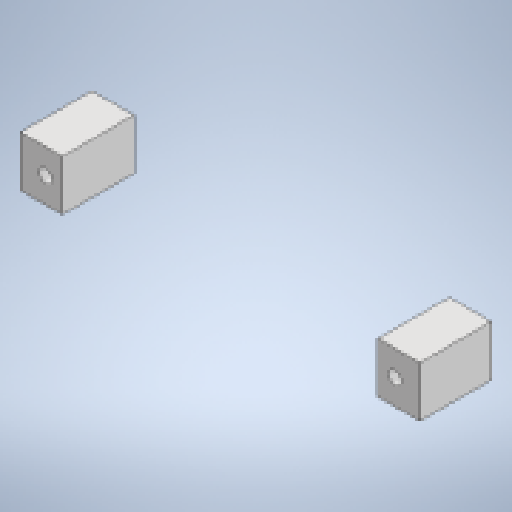
# Autodesk Inventor part: Tapadera cremallera
Saved by Autodesk Inventor 2024 (Build 280153000, 153)
## iProperties
Created: 2025-03-05
Part Number: Tapadera cremallera
Material: Genérico
Document SubType Name: Modeling
Designer: sergi
Density: 1 g/cm^3
Appearance: Valor por defecto
Author: sergi
Autodesk Inventor part; units mm, degrees
ref_plane "YZ Plane" through (0, 0, 0) normal (1, 0, 0) x (0, 1, 0)
ref_plane "XZ Plane" through (0, 0, 0) normal (0, 1, 0) x (-1, 0, 0)
sketch "Boceto1" plane through (0, 0, 0) normal (0, 0, 1) x (1, 0, 0)
  line L0 (9.8963, 1.0011) -> (-9.8944, 1.0011) projected
  arc A0 (-33.0611, -12.6806) -> (-9.8944, 1.0011) centre (-23.4499, -2.5004) ccw projected
  line L1 (-33.0611, -12.6806) -> (-33.2, -12.6806) projected
  line L2 (-33.2, -12.6806) -> (-33.2, -12.5477) projected
  arc A1 (-37.0054, 1.0011) -> (-33.2, -12.5477) centre (-23.4499, -2.5004) ccw projected
  line L3 (-37.0054, 1.0011) -> (-47.5, 1.0011) projected
  line L4 (-47.5, 1.0011) -> (-47.5, -20) projected
  line L5 (-47.5, -20) -> (47.5, -20) projected
  line L6 (47.5, -20) -> (47.5, 1.0011) projected
  line L7 (47.5, 1.0011) -> (37.0052, 1.0011) projected
  arc A2 (33.2, -12.5466) -> (37.0052, 1.0011) centre (23.4507, -2.5001) ccw projected
  line L8 (33.2, -12.5466) -> (33.2, -12.6806) projected
  line L9 (33.2, -12.6806) -> (33.06, -12.6806) projected
  arc A3 (9.8963, 1.0011) -> (33.06, -12.6806) centre (23.4507, -2.5001) ccw projected
  circle A4 centre (40.9504, -2.4989) radius 2.1 projected
  circle A5 centre (5.9501, -2.5002) radius 2.1 projected
  circle A6 centre (-5.9495, -2.4989) radius 2.1 projected
  circle A7 centre (-40.9494, -2.4994) radius 2.1 projected
  line L10 (47.5, -20) -> (41.5, -20)
  line L11 (41.5, -20) -> (41.5, -14)
  line L12 (41.5, -14) -> (47.5, -14)
  line L13 (47.5, -14) -> (47.5, -20)
  circle A8 centre (41.5, -14) radius 1.6
  line L14 (-47.5, -20) -> (-41.5, -20)
  line L15 (-41.5, -20) -> (-41.5, -14)
  line L16 (-41.5, -14) -> (-47.5, -14)
  line L17 (-47.5, -14) -> (-47.5, -20)
  circle A9 centre (-41.5, -14) radius 1.6
  line L18 (47.5, -20) -> (33.5, -20)
  line L19 (33.5, -20) -> (33.5, -8)
  line L20 (33.5, -8) -> (47.5, -8)
  line L21 (47.5, -8) -> (47.5, -20)
  line L22 (-47.5, -20) -> (-33.5, -20)
  line L23 (-33.5, -20) -> (-33.5, -8)
  line L24 (-33.5, -8) -> (-47.5, -8)
  line L25 (-47.5, -8) -> (-47.5, -20)
  line L26 (33.2, -20.6806) -> (-33.2, -20.6806) projected
  line L27 (33.2, -12.6806) -> (33.2, -20.6806) projected
  line L28 (33.2, -12.6806) -> (30.95, -12.6806) projected
  arc A10 (25.95, -17.6806) -> (30.95, -12.6806) centre (25.95, -12.6806) ccw projected
  line L29 (25.95, -17.6806) -> (-25.95, -17.6806) projected
  arc A11 (-30.95, -12.6806) -> (-25.95, -17.6806) centre (-25.95, -12.6806) ccw projected
  line L30 (-33.2, -12.6806) -> (-30.95, -12.6806) projected
  line L31 (-33.2, -20.6806) -> (-33.2, -12.6806) projected
  line L32 (33.2, 62.3194) -> (33.2, -12.6806)
  line L33 (-33.2, -12.6806) -> (-33.2, 62.3194)
  circle A12 centre (-41.5, -14) radius 2.1 projected
  circle A13 centre (41.5, -14) radius 2.1 projected
  point P0 (0, 0)
  point P1 (47.5, -8)
  point P2 (33.5, -20)
  point P3 (-33.5, -20)
  point P4 (-47.5, -8)
  point P5 (-33.5, -12.2476)
  point P6 (-36.3249, -8)
  point P7 (36.3244, -8)
  point P8 (33.5, -12.2466)
  dimension "d0" = 6
  dimension "d1" = 6
  dimension "d2" = 3.2
  dimension "d3" = 6
  dimension "d4" = 6
  dimension "d5" = 3.2
  dimension "d6" = 14
  dimension "d7" = 12
  dimension "d8" = 14
  dimension "d9" = 12
  constraints: 36 end point, 8 parallel, 4 horizontal, 4 perpendicular, 2 centre point, 2 coincident, 2 vertical, 6 other
  measures "d0" distance of L11.end L12.end
  measures "d1" distance of L10.end L11.end
  measures "d2" diameter of A8
  measures "d3" distance of L16.end L15.end
  measures "d4" distance of L15.end L14.end
  measures "d5" diameter of A9
  measures "d6" distance of L19.end L20.end
  measures "d7" distance of L18.end L19.end
  measures "d8" distance of L24.end L23.end
  measures "d9" distance of L23.end L22.end
ref_plane "Plano de trabajo1" through (-47.5, -94.8095, 26) normal (0, 0, 1) x (1, 0.0000001, 0)
extrude "Extrusión1" add sketch "Boceto1" along normal blind 17 contours A2 L20 L6 L12 A13 L11 L5 L19 | L23 L5 L15 A12 L16 L4 L24 A1 | L11 A13 L12 L6 L5 | L5 L4 L16 A12 L15 | A13 L12 A8 L11 | L11 A8 L12 A13 | A12 L16 A9 L15 | L15 A9 L16 A12
sketch "Boceto2" plane through (33.5, -20, 0) normal (-1, 0, 0) x (0, 0, 1)
  line L0 (0, 7.7534) -> (0, 0) projected
  line L1 (0, 0) -> (17, 0) projected
  line L2 (17, 7.7534) -> (17, 0) projected
  line L3 (0, 7.7534) -> (17, 7.7534) projected
  line L4 (13, 7.3194) -> (13, -0.6806) projected
  line L5 (13.6, 7.7534) -> (13.6, -0.6806)
  line L6 (0, 12) -> (0, 7.7534) projected
  line L7 (0, 7.7534) -> (17, 7.7534) projected
  line L8 (17, 12) -> (17, 7.7534) projected
  line L9 (0, 12) -> (17, 12) projected
  line L10 (13.6, 0) -> (17, 0)
  line L11 (17, 0) -> (17, 35)
  line L12 (17, 35) -> (13.6, 35)
  line L13 (13.6, 35) -> (13.6, 0)
  point P0 (0, 20)
  point P1 (17, 7.7534)
  point P2 (17, 12)
  point P3 (13.6, 12)
  point P4 (17, 12)
  point P5 (0, 7.7534)
  point P6 (17, 7.7534)
  point P7 (17, 7.7534)
  point P8 (13.6, 7.7534)
  point P9 (0, 7.7534)
  point P10 (17, 7.7534)
  point P11 (0, 7.7534)
  dimension "d12" = 0.6
  dimension "d13" = 35
  constraints: 10 end point, 3 parallel, 3 point on line, 1 horizontal, 1 perpendicular
  measures "d12" distance between parallel lines of L4 L5
  measures "d13" distance of L11.end L10.end
extrude "Extrusión2" add sketch "Boceto2" along normal blind 72 and the other way blind 5 contours L13 L9 L8 L3 | L3 L2 L1 L5 | L13 L12 L11 L9
sketch "Boceto3" plane through (33.5, -20, 13.6) normal (0, 0, -1) x (-1, 0, 0)
  line L0 (67, 7.7524) -> (67, 0) projected
  arc A0 (67, 7.7524) -> (69.8249, 12) centre (56.9499, 17.4996) ccw projected
  line L1 (72, 12) -> (69.8249, 12) projected
  line L2 (72, 35) -> (72, 12) projected
  line L3 (72, 35) -> (-5, 35) projected
  line L4 (-5, 12) -> (-5, 35) projected
  line L5 (-2.8244, 12) -> (-5, 12) projected
  arc A1 (-2.8244, 12) -> (0, 7.7534) centre (10.0493, 17.4999) ccw projected
  line L6 (0, 0) -> (0, 7.7534) projected
  line L7 (0, 0) -> (67, 0) projected
  line L8 (0.3, 7.3194) -> (0.3, 82.3194) projected
  line L9 (0, 7.7534) -> (0.3, 7.7534)
  line L10 (66.7, 7.3194) -> (66.7, 82.3194) projected
  line L11 (67, 7.7524) -> (67, 0) projected
  line L12 (67, 7.7524) -> (67, 36)
  line L13 (0, 7.7534) -> (0, 35.331)
  point P0 (33.5, 20)
  point P1 (0.3, 35)
  point P2 (67, 35)
  point P3 (0, 35)
  constraints: 6 end point, 2 perpendicular, 1 horizontal, 1 point on line
extrude "Extrusión3" add sketch "Boceto3" along normal blind 9.6 contours L12 L3 L2 L1 A0 | A1 L5 L4 L3 L13
